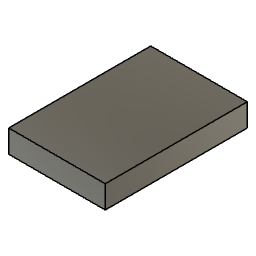
controller v1 (Autodesk Fusion 360 archive; units mm, degrees)
design "battery 803450"
Autodesk Fusion 360 part; units mm, degrees
sketch "Sketch1" plane through (0, 0, 0) normal (0, 0, 1) x (1, 0, 0)
  line L0 (17, 25) -> (-17, 25)
  line L1 (-17, 25) -> (-17, -25)
  line L2 (-17, -25) -> (17, -25)
  line L3 (17, -25) -> (17, 25)
  line L4 (17, 25) -> (-17, -25) construction
  line L5 (-17, 25) -> (17, -25) construction
  dimension "d1" = 34
  constraint horizontal L0
  constraint perpendicular L0 L1
  constraint parallel L0 L2
  constraint parallel L1 L3
  constraint coincident L4 origin
  constraint coincident L5 origin
  measures "d1" distance of L1.end L2.end
extrude "Extrude1" add sketch "Sketch1" along normal blind 8
